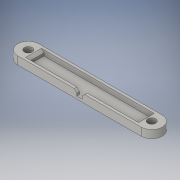
# Autodesk Inventor part: Beaglebone Antenna Mount
Saved by Autodesk Inventor 2016 (Build 200138000, 138)
## iProperties
Created: 2016-06-22
Part Number: Beaglebone Antenna Mount
Material: Generic
Document SubType Name: Modeling
Designer: Jacob
Density: 1 g/cm^3
Appearance: Default
Author: Jacob
Autodesk Inventor part; units mm, degrees
ref_plane "YZ Plane" through (0, 0, 0) normal (1, 0, 0) x (0, 1, 0)
ref_plane "XZ Plane" through (0, 0, 0) normal (0, 1, 0) x (-1, 0, 0)
ref_plane "XY Plane" through (0, 0, 0) normal (0, 0, 1) x (1, 0, 0)
sketch "Sketch1" plane through (0, 0, 0) normal (0, 1, 0) x (-1, 0, 0)
  line L0 (0, 0) -> (6, 0)
  line L1 (6, 0) -> (6, -41)
  line L2 (6, -41) -> (0, -41)
  line L3 (0, -41) -> (0, 0)
  line L4 (7, -42) -> (7, 1)
  line L5 (7, 1) -> (-1, 1)
  line L6 (-1, 1) -> (-1, -42)
  line L7 (-1, -42) -> (7, -42)
  line L8 (3, 1) -> (3, 3)
  circle A0 centre (3, 3) radius 1.5
  arc A1 (7, 3) -> (-1, 3) centre (3, 3) ccw
  line L9 (7, 1) -> (7, 3)
  line L10 (-1, 1) -> (-1, 3)
  line L11 (3, -42) -> (3, -44)
  circle A2 centre (3, -44) radius 1.5
  arc A3 (-1, -44) -> (7, -44) centre (3, -44) ccw
  line L12 (7, -42) -> (7, -44)
  line L13 (-1, -42) -> (-1, -44)
  dimension "d19" = 2
  dimension "d0" = 6
  dimension "d1" = 41
  dimension "d2" = 1
  dimension "d3" = 2
  dimension "d4" = 3
  dimension "d5" = 8
  dimension "d6" = 2
  dimension "d7" = 3
  dimension "d8" = 8
  constraints: 28 end point, 4 centre point, 4 coincident, 4 parallel, 4 point on circle, 4 tangent, 2 midpoint, 2 perpendicular, 2 vertical, 1 horizontal, 3 other
  measures "d0" distance of L1.end L2.end
  measures "d1" distance of L0.end L1.end
  measures "d2" distance between parallel lines of L1 L4
  measures "d3" distance of L8.start L8.end
  measures "d4" diameter of A0
  measures "d5" diameter of A1
  measures "d6" distance of L11.start L11.end
  measures "d7" diameter of A2
  measures "d8" diameter of A3
extrude "Extrusion1" add sketch "Sketch1" along normal blind 3
sketch "Sketch2" plane through (0, 3, 0) normal (0, 1, 0) x (1, 0, 0)
  line L0 (0, 41) -> (0, 0) projected
  line L1 (-6, 0) -> (-6, 41) projected
  line L2 (0, 0) -> (-6, 0)
  line L3 (-6, 0) -> (-6, 41)
  line L4 (-6, 41) -> (0, 41)
  line L5 (0, 41) -> (0, 0)
  constraints: 8 end point, 2 parallel, 1 horizontal, 1 perpendicular
extrude "Extrusion2" add sketch "Sketch2" against normal blind 1
sketch "Sketch3" plane through (0, 0, 0) normal (0, -1, 0) x (1, 0, 0)
  circle A0 centre (-3, 3) radius 1.5 projected
  line L0 (-6, -41) -> (-6, 0) projected
  line L1 (-6, 0) -> (0, 0) projected
  line L2 (0, 0) -> (0, -41) projected
  line L3 (0, -41) -> (-6, -41) projected
  circle A1 centre (-3, 3) radius 1.5 projected
  circle A2 centre (-3, -44) radius 1.5 projected
  line L4 (-7, -44) -> (-7, 3) projected
  arc A3 (-7, -44) -> (1, -44) centre (-3, -44) ccw projected
  line L5 (1, 3) -> (1, -44) projected
  arc A4 (1, 3) -> (-7, 3) centre (-3, 3) ccw projected
  line L6 (-7, -44) -> (-7, 3) projected
  line L7 (-7, -20.5) -> (-7, -21.5)
  line L8 (-7, -21.5) -> (-6, -21.5)
  line L9 (-6, -21.5) -> (-6, -19.5)
  line L10 (-6, -19.5) -> (-7, -19.5)
  line L11 (-7, -19.5) -> (-7, -21.5)
  dimension "d13" = 1
  dimension "d14" = 1
  dimension "d15" = 2
  constraints: 10 end point, 2 parallel, 1 horizontal, 1 midpoint, 1 perpendicular, 1 point on line
  measures "d13" distance of L7.start L7.end
  measures "d14" distance of L10.end L9.end
  measures "d15" distance of L9.end L8.end
extrude "Extrusion3" cut sketch "Sketch3" against normal up to surface (2 mm away) contours L8 L4 L10 L0
chamfer "Chamfer1" distance 1 angle 45 2 edges at (-6.5, 0, -19.5) (-6.5, 0, -21.5)
chamfer "Chamfer2" distance 1 angle 45 2 edges at (-3, 0, 0) (-3, 0, -41)
body "Solid1"
